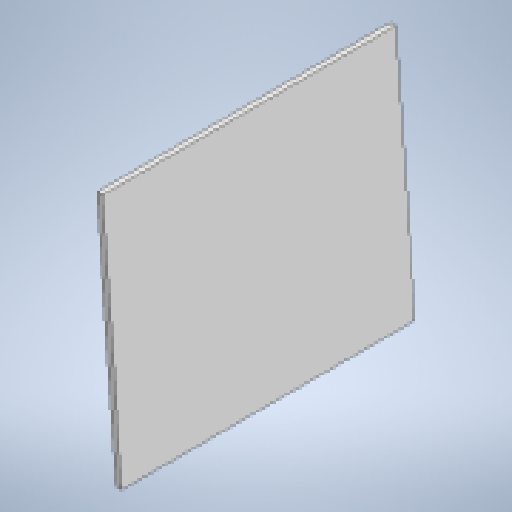
# Autodesk Inventor part: szkic
Saved by Autodesk Inventor 2023 (Build 270158000, 158)
## iProperties
Created: 2023-08-22
Part Number: szkic
Material: Ogólny
Document SubType Name: Modeling
Designer: Kamil
Density: 1 g/cm^3
Appearance: Domyślna
Author: Kamil
Autodesk Inventor part; units mm, degrees
ref_plane "YZ Plane" through (0, 0, 0) normal (1, 0, 0) x (0, 1, 0)
ref_plane "XZ Plane" through (0, 0, 0) normal (0, 1, 0) x (-1, 0, 0)
ref_plane "XY Plane" through (0, 0, 0) normal (0, 0, 1) x (1, 0, 0)
sketch "Szkic1" plane through (0, 0, 0) normal (0, 0, 1) x (1, 0, 0)
  circle A0 centre (0, 0) radius 15 projected
  line L0 (-8.4451, -84.98) -> (-14.955, -1.1615)
  line L1 (-10.4511, -84.98) -> (-16.949, -1.3164)
  line L2 (-8.4451, -84.98) -> (-10.4511, -84.98)
  line L3 (-14.955, -1.1615) -> (-16.949, -1.3164)
  line L4 (-8.4451, -84.98) -> (-16.1884, 14.7198)
  line L5 (-16.1884, 14.7198) -> (19.05, 17.4566)
  line L6 (0, 0) -> (-1.2334, 15.8813)
  line L7 (-1.1615, 14.955) -> (-1.2334, 15.8813)
  point P0 (0, 0)
  dimension "d0" = 2
  dimension "d1" = 100
  constraints: 16 end point, 3 perpendicular, 2 parallel, 2 point on circle, 2 point on line, 1 collinear, 1 horizontal, 1 tangent, 1 other
  measures "d0" distance between parallel lines of L0 L1
  measures "d1" distance of L0.start L4.end
extrude "Wyciągnięcie proste1" add sketch "Szkic1" along normal blind 4.8 and the other way blind 95.2 contours L0 L2 L1 L3
